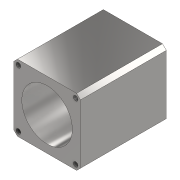
# Autodesk Inventor part: Cover for servo motor 250 W
Saved by Autodesk Inventor 2020.3 (Build 243373010, 373A)
## iProperties
Created: 2021-04-26
Part Number: Cover for servo motor 250 W
Material: Stainless Steel
Document SubType Name: Modeling
Designer: marti
Density: 8 g/cm^3
Appearance: Semi-Polished
Author: marti
Autodesk Inventor part; units mm, degrees
ref_plane "YZ Plane" through (0, 0, 0) normal (1, 0, 0) x (0, 1, 0)
ref_plane "XZ Plane" through (0, 0, 0) normal (0, 1, 0) x (-1, 0, 0)
ref_plane "XY Plane" through (0, 0, 0) normal (0, 0, 1) x (1, 0, 0)
sketch "Sketch1" plane through (0, 0, 0) normal (0, 0, 1) x (1, 0, 0)
  line L0 (-17.5, 17.5) -> (17.5, 17.5)
  line L1 (17.5, 17.5) -> (17.5, -17.5)
  line L2 (17.5, -17.5) -> (-17.5, -17.5)
  line L3 (-17.5, -17.5) -> (-17.5, 17.5)
  line L4 (14.5, 14.5) -> (-14.5, 14.5)
  line L5 (-14.5, 14.5) -> (-14.5, -14.5)
  line L6 (-14.5, -14.5) -> (14.5, -14.5)
  line L7 (14.5, -14.5) -> (14.5, 14.5)
  point P0 (0, 0)
  point P1 (17.5, 0)
  point P2 (0, 17.5)
  dimension "d0" = 35
  dimension "d1" = 35
  dimension "d2" = 3
  constraints: 16 end point, 4 parallel, 2 midpoint, 2 perpendicular, 1 horizontal, 1 horizontal alignment, 1 vertical alignment, 3 other
  measures "d0" distance of L0.end L1.end
  measures "d1" distance of L0.start L0.end
  measures "d2" distance between parallel lines of L0 L4
extrude "Extrusion1" add sketch "Sketch1" against normal mid plane 45
chamfer "Chamfer1" distance 2 angle 45 8 edges at (-17.5, 17.5, 0) (17.5, 17.5, 0) (-14.5, 14.5, 0) (14.5, 14.5, 0) (-14.5, -14.5, 0) (14.5, -14.5, 0) (17.5, -17.5, 0) (-17.5, -17.5, 0)
sketch "Sketch2" plane through (0, 0, 22.5) normal (0, 0, 1) x (1, 0, 0)
  line L0 (15.5, 17.5) -> (-15.5, 17.5) projected
  line L1 (-12.5, 14.5) -> (12.5, 14.5) projected
  line L2 (-17.5, 15.5) -> (-15.5, 17.5) projected
  line L3 (-12.5, 14.5) -> (-14.5, 12.5) projected
  line L4 (14.5, 12.5) -> (12.5, 14.5) projected
  line L5 (15.5, 17.5) -> (17.5, 15.5) projected
  line L6 (-17.5, 15.5) -> (-17.5, -15.5) projected
  line L7 (-14.5, -12.5) -> (-14.5, 12.5) projected
  line L8 (-14.5, -12.5) -> (-12.5, -14.5) projected
  line L9 (-15.5, -17.5) -> (15.5, -17.5) projected
  line L10 (17.5, -15.5) -> (17.5, 15.5) projected
  line L11 (-15.5, -17.5) -> (-17.5, -15.5) projected
  line L12 (12.5, -14.5) -> (-12.5, -14.5) projected
  point P0 (0, 0)
  point P1 (-15, 15)
  point P2 (15, 15)
  point P3 (15, -15)
  point P4 (-15, -17.5)
  point P5 (-15, -15)
  point P6 (15, -17.5)
  dimension "d8" = 3
  dimension "d9" = 4.2426
  dimension "d10" = 2.1213
  dimension "d11" = 5
  dimension "d12" = 2.5
  dimension "d13" = 2.5
  dimension "d14" = 4.2426
  dimension "d15" = 2.1213
  dimension "d26" = 5
  dimension "d27" = 2.5
  dimension "d28" = 5
  dimension "d29" = 2.5
  dimension "d30" = 2.5
  dimension "d31" = 2.5
  dimension "d64" = 4.2426
  constraints: 2 other
  measures "d8" distance between parallel lines of L0 L1
  measures "d9" distance between parallel lines of L2 L3
  measures "d10" distance from line of L2 point (-15, 15)
  measures "d11" vertical distance of L3.end L0.end
  measures "d12" vertical distance of L0.end point (-15, 15)
  measures "d13" vertical distance of L0.start point (15, 15)
  measures "d14" distance between parallel lines of L4 L5
  measures "d15" distance from line of L4 point (15, 15)
  measures "d28" distance from line of L9 L7.start
  measures "d29" distance from line of L9 point (-15, -15)
  measures "d30" distance from line of L9 point (15, -15)
  measures "d64" distance between parallel lines of L11 L8
hole "Hole1" at (-15, 15, 22.5) at (15, 15, 22.5) at (15, -15, 22.5) at (-15, -15, 22.5) direction (0, 0, -1) diameter 2.459 depth 8.8 tip angle 118 thread size "M3x0.5" class "6H" standard "ISO Metric profile"
sketch "Sketch4" plane through (0, 0, -22.5) normal (0, 0, -1) x (-1, 0, 0)
  line L0 (15.5, 17.5) -> (-15.5, 17.5)
  line L1 (-12.5, 14.5) -> (12.5, 14.5)
  line L2 (-17.5, 15.5) -> (-15.5, 17.5)
  line L3 (-12.5, 14.5) -> (-14.5, 12.5)
  line L4 (14.5, 12.5) -> (12.5, 14.5)
  line L5 (15.5, 17.5) -> (17.5, 15.5)
  line L6 (-17.5, 15.5) -> (-17.5, -17.5)
  line L7 (-14.5, -12.5) -> (-14.5, 12.5)
  line L8 (-14.5, -12.5) -> (-12.5, -14.5)
  line L9 (-17.5, -17.5) -> (17.5, -17.5)
  line L10 (17.5, -17.5) -> (17.5, 15.5)
  line L11 (-17.5, 15.5) -> (-15.5, 17.5) projected
  line L12 (-17.5, 15.5) -> (-17.5, -15.5) projected
  line L13 (-15.5, -17.5) -> (15.5, -17.5) projected
  line L14 (17.5, -15.5) -> (17.5, 15.5) projected
  line L15 (15.5, 17.5) -> (17.5, 15.5) projected
  line L16 (15.5, 17.5) -> (-15.5, 17.5) projected
  line L17 (-14.5, -12.5) -> (-14.5, 12.5) projected
  line L18 (-12.5, 14.5) -> (-14.5, 12.5) projected
  line L19 (-12.5, 14.5) -> (12.5, 14.5) projected
  line L20 (14.5, 12.5) -> (12.5, 14.5) projected
  line L21 (14.5, 12.5) -> (14.5, -12.5) projected
  line L22 (12.5, -14.5) -> (14.5, -12.5) projected
  line L23 (12.5, -14.5) -> (-12.5, -14.5) projected
  line L24 (-14.5, -12.5) -> (-12.5, -14.5) projected
  line L25 (17.5, -15.5) -> (15.5, -17.5) projected
  line L26 (-15.5, -17.5) -> (-17.5, -15.5) projected
  point P0 (0, 0)
  point P1 (0, 0)
  point P2 (-15, 15)
  point P3 (15, 15)
  point P4 (15, -15)
  point P5 (-15, -15)
  dimension "d39" = 3
  dimension "d40" = 4.2426
  dimension "d41" = 2.1213
  dimension "d42" = 5
  dimension "d43" = 2.5
  dimension "d44" = 2.5
  dimension "d45" = 4.2426
  dimension "d46" = 2.1213
  dimension "d47" = 5.6569
  dimension "d48" = 5
  dimension "d49" = 2.5
  dimension "d50" = 5
  dimension "d51" = 2.5
  dimension "d52" = 2.5
  dimension "d53" = 2.5
  constraints: 22 end point
  measures "d39" distance between parallel lines of L0 L1
  measures "d40" distance between parallel lines of L2 L3
  measures "d41" distance from line of L2 point (-15, 15)
  measures "d42" vertical distance of L0.end L3.end
  measures "d43" vertical distance of L0.end point (-15, 15)
  measures "d44" vertical distance of L0.start point (15, 15)
  measures "d45" distance between parallel lines of L4 L5
  measures "d46" distance from line of L4 point (15, 15)
  measures "d47" distance from line of L6.end L8
  measures "d48" distance from line of L8.end L6
  measures "d49" distance from line of L6 point (-15, -15)
  measures "d50" distance from line of L7.start L9
  measures "d51" distance from line of L9 point (-15, -15)
  measures "d52" distance from line of L9 point (15, -15)
  measures "d53" distance from line of L10 point (15, -15)
hole "Hole2" at (15, 15, -22.5) at (-15, 15, -22.5) at (-15, -15, -22.5) at (15, -15, -22.5) direction (0, 0, 1) diameter 2.459 depth 8.8 tip angle 118 thread size "M3x0.5" class "6H" standard "ISO Metric profile"
sketch "Sketch7" plane through (0, 0, 22.5) normal (0, 0, 1) x (1, 0, 0)
  circle A0 centre (0, 0) radius 13.25
  circle A1 centre (15, -15) radius 1.2295 projected
  circle A2 centre (-15, 15) radius 1.2295 projected
  circle A3 centre (15, 15) radius 1.2295 projected
  circle A4 centre (-15, -15) radius 1.2295 projected
  line L0 (15.5, 17.5) -> (17.5, 15.5) projected
  line L1 (15.5, 17.5) -> (-15.5, 17.5) projected
  line L2 (-17.5, 15.5) -> (-15.5, 17.5) projected
  line L3 (-17.5, 15.5) -> (-17.5, -15.5) projected
  line L4 (-15.5, -17.5) -> (15.5, -17.5) projected
  line L5 (17.5, -15.5) -> (17.5, 15.5) projected
  line L6 (14.5, 12.5) -> (14.5, -12.5) projected
  line L7 (12.5, -14.5) -> (14.5, -12.5) projected
  line L8 (12.5, -14.5) -> (-12.5, -14.5) projected
  line L9 (-14.5, -12.5) -> (-12.5, -14.5) projected
  line L10 (-14.5, -12.5) -> (-14.5, 12.5) projected
  line L11 (-12.5, 14.5) -> (-14.5, 12.5) projected
  line L12 (-12.5, 14.5) -> (12.5, 14.5) projected
  line L13 (14.5, 12.5) -> (12.5, 14.5) projected
  line L14 (-15.5, -17.5) -> (-17.5, -15.5) projected
  line L15 (17.5, -15.5) -> (15.5, -17.5) projected
  dimension "d61" = 26.5
  constraints: 1 centre point, 1 coincident
  measures "d61" diameter of A0
extrude "Extrusion2" add sketch "Sketch7" against normal blind 35 contours L6 L7 L8 L9 L10 L11 L12 L13
equation "\"d10\" = 0.5 * d9"
equation "\"d12\" = 0.5 * d11"
equation "\"d13\" = d12"
equation "\"d15\" = d10"
equation "\"d27\" = 0.5 * d26"
equation "\"d29\" = 0.5 * d28"
equation "\"d30\" = d29"
equation "\"d31\" = d27"
equation "\"d41\" = 0.5 * d40"
equation "\"d43\" = 0.5 * d42"
equation "\"d44\" = d43"
equation "\"d46\" = d41"
equation "\"d49\" = 0.5 * d48"
equation "\"d51\" = 0.5 * d50"
equation "\"d52\" = d51"
equation "\"d53\" = d49"
body "Solid1"
